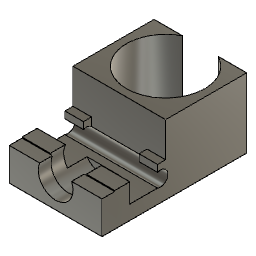
Radiator_Holder_Version_2 (Autodesk Fusion 360 design; units mm, degrees)
Autodesk Fusion 360 part; units mm, degrees
note: some values were not read from the file. Set by a fixed rule: which sketch regions a step uses.
sketch "Main Body" plane through (0, 0, 0) normal (0, 0, 1) x (1, 0, 0)
  circle A0 centre (0, 0) radius 16.85
  line L0 (-20, 20) -> (20, 20)
  line L1 (20, 20) -> (20, -20)
  line L2 (20, -20) -> (-20, -20)
  line L3 (-20, -20) -> (-20, 20)
  line L4 (-20, 15) -> (20, 15)
  point P0 (-20, 0)
  point P1 (0, 20)
  dimension "d1" = 33.7
  dimension "d2" = 40
  dimension "d3" = 15
  constraint coincident A0.centre origin
  constraint horizontal L0
  constraint vertical L1
  constraint horizontal L2
  constraint vertical L3
  constraint equal L0 L3
  constraint midpoint L3 P0
  constraint midpoint L0 P1
  constraint vertical A0.centre P1
  constraint horizontal A0.centre P0
  constraint coincident L3 L4.start
  constraint coincident L1 L4.end
  constraint perpendicular L1 L4
  measures "d1" diameter of A0
  measures "d2" distance of L0.start L2.end
  measures "d3" distance of A0.centre L4
extrude "Extrude1" add sketch "Main Body" along normal blind 30 contours A0 L1 L2 L3 L4
sketch "Antenna Holder" plane through (20, 0, 0) normal (1, 0, 0) x (0, 1, 0)
  line L0 (-20, 0) -> (15, 0)
  line L1 (15, 0) -> (15, 30)
  line L2 (15, 30) -> (-20, 30)
  line L3 (-20, 30) -> (-20, 0)
  circle A0 centre (-22.2, 9.1) radius 3.2
  line L4 (-23.48, 15) -> (-20, 15)
  line L5 (-20, 15) -> (-20, 0)
  line L6 (-20, 0) -> (-23.48, 0)
  line L7 (-23.48, 0) -> (-23.48, 15)
  point P0 (-23.48, 6.1672)
  dimension "d6" = 6.4
  dimension "d7" = 22.2
  dimension "d8" = 20.9
  dimension "d9" = 1.28
  constraint horizontal L4
  constraint vertical L5
  constraint horizontal L6
  constraint vertical L7
  constraint collinear L3 L5
  constraint collinear L0 L6
  constraint coincident A0 P0
  constraint coincident L7 P0
  measures "d6" diameter of A0
  measures "d7" horizontal distance of origin A0.centre
  measures "d8" distance of L2 A0.centre
  measures "d9" distance of A0.centre L7
extrude "Extrude2" add sketch "Antenna Holder" against normal blind 40 contours L3 A0 L5 L6 L7 | L3 A0 L5 | L3 A0 L4 L5 L7
extrude "Extrude3" cut sketch "Antenna Holder" against normal blind 40 contours L3 A0 L5
sketch "Coax_Connector_holder" plane through (20, -21.74, 3.3881) normal (1, 0, 0) x (0, 1, 0)
  line L0 (-1.74, 2.779) -> (-13.74, 2.779)
  line L1 (-13.74, 2.779) -> (-13.74, -3.3881)
  line L2 (-13.74, -3.3881) -> (-1.74, -3.3881)
  line L3 (-1.74, -3.3881) -> (-1.74, 2.779)
  line L4 (1.74, -3.3881) -> (36.74, -3.3881)
  line L5 (-1.74, -3.3881) -> (-1.74, 11.6119)
  line L6 (-13.74, -3.3881) -> (-25.74, -3.3881)
  line L7 (-25.74, -3.3881) -> (-25.74, 11.6119)
  line L8 (-25.74, 11.6119) -> (-13.74, 11.6119)
  line L9 (-13.74, 11.6119) -> (-13.74, -3.3881)
  line L10 (-1.74, 11.6119) -> (1.74, 11.6119)
  point P0 (-1.74, 2.779)
  point P1 (-0.46, 5.7119)
  dimension "d15" = 12
  dimension "d16" = 12
  constraint horizontal L0
  constraint vertical L1
  constraint horizontal L2
  constraint vertical L3
  constraint collinear L2 L4
  constraint collinear L3 L5
  constraint coincident L0 P0
  constraint horizontal L6
  constraint vertical L7
  constraint vertical L9
  constraint collinear L1 L9
  constraint collinear L8 L10
  constraint collinear L2 L6
  measures "d15" distance of L1.end L2.end
  measures "d16" distance of L1.end L6.end
extrude "Extrude4" add sketch "Coax_Connector_holder" against normal blind 40
sketch "Connector_Hole" plane through (0, -47.48, 0) normal (0, -1, 0) x (1, 0, 0)
  line L0 (20, 0) -> (20, 15)
  line L1 (20, 15) -> (-20, 15)
  line L2 (-20, 15) -> (-20, 0)
  line L3 (-20, 0) -> (20, 0)
  circle A0 centre (0, 11.1) radius 7.5
  circle A1 centre (0, 11.1) radius 8.5
  line L4 (-20, 30) -> (20, 30)
  line L5 (-20, 14.1) -> (20, 14.1)
  line L6 (-20, 14.5) -> (20, 14.5)
  dimension "d19" = 17
  dimension "d20" = 15
  dimension "d21" = 18.9
  dimension "d22" = 3
  dimension "d23" = 3.4
  constraint concentric A0 A1
  constraint vertical origin A0.centre
  constraint coincident L2 L5.start
  constraint coincident L0 L5.end
  constraint perpendicular L0 L5
  constraint coincident L2 L6.start
  constraint perpendicular L2 L6
  measures "d19" diameter of A1
  measures "d20" diameter of A0
  measures "d21" distance of A0.centre L4
  measures "d22" distance of A0.centre L5
  measures "d23" distance of A0.centre L6
extrude "Extrude5" cut sketch "Connector_Hole" against normal blind 5.5 contours L0 A1 L5 L6 | L0 L1 A1 L6 | A0 A1 L5 L6 | L2 A1 L5 L6 | L1 A0 A1 L6 | A0 L5 L6 | A0 L5 | L1 L2 A1 L6 | A0 A1 L5 L6 | L1 A0 L6 | L1 A0 A1 L6
extrude "Extrude6" cut sketch "Connector_Hole" against normal blind 15 from surface at -5.5 contours L0 L1 A1 L6 | A0 A1 L5 L6 | A0 A1 L5 | L1 A0 A1 L6 | A0 L5 L6 | A0 L5 | L1 L2 A1 L6 | A0 A1 L5 L6 | L1 A0 L6 | L1 A0 A1 L6
sketch "Sketch5" plane through (0, 0, 15) normal (0, 0, 1) x (-1, 0, 0)
  line L0 (-20, 23.48) -> (-20, 20)
  line L1 (-20, 20) -> (20, 20)
  line L2 (20, 20) -> (20, 23.48)
  line L3 (20, 23.48) -> (-20, 23.48)
  line L4 (12, 20) -> (12, 23.48)
  line L5 (-12, 20) -> (-12, 23.48)
  dimension "d29" = 8
  dimension "d30" = 8
  constraint coincident L1 L4.start
  constraint coincident L3 L4.end
  constraint perpendicular L3 L4
  constraint coincident L1 L5.start
  constraint coincident L3 L5.end
  constraint perpendicular L3 L5
  measures "d29" distance of L2 L4
  measures "d30" distance of L0 L5
extrude "Extrude7" cut sketch "Sketch5" against normal blind 5 contours L1 L3 L4 L5
equation "d7 = 19 mm + 3.2 mm"
equation "d9 = d6 / 5"
equation "d10 = -d2"
equation "d12 = -d2"
equation "d17 = -d2"
equation "d21 = d8 - 2 mm"
equation "d22 = d20 / 5"
equation "d23 = d19 / 5"
